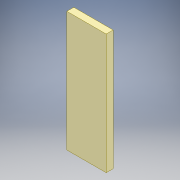
# Autodesk Inventor part: 51单片机
Saved by Autodesk Inventor 2018 (Build 220112000, 112)
## iProperties
Created: 2020-11-25
Part Number: 51单片机
Material: 尼龙 6/6
Document SubType Name: Modeling
Designer: OHHHHHHHHHH
Density: 1.13 g/cm^3
Appearance: 尼龙 6
Author: OHHHHHHHHHH
Autodesk Inventor part; units mm, degrees
ref_plane "YZ Plane" through (0, 0, 0) normal (1, 0, 0) x (0, 1, 0)
ref_plane "XZ Plane" through (0, 0, 0) normal (0, 1, 0) x (-1, 0, 0)
ref_plane "XY Plane" through (0, 0, 0) normal (0, 0, 1) x (1, 0, 0)
sketch "草图1" plane through (0, 0, 0) normal (0, 1, 0) x (-1, 0, 0)
  line L0 (0, 0) -> (17, 0)
  line L1 (17, 0) -> (17, -52)
  line L2 (17, -52) -> (0, -52)
  line L3 (0, -52) -> (0, 0)
  dimension "d0" = 52
  dimension "d1" = 17
  constraints: 8 end point, 2 parallel, 1 horizontal, 1 perpendicular
  measures "d0" distance of L0.end L1.end
  measures "d1" distance of L0.start L0.end
extrude "拉伸1" add sketch "草图1" along normal blind 3
sketch "草图2" plane through (0, 3, 0) normal (0, 1, 0) x (1, 0, 0)
  line L0 (-8.4489, 20.8819) -> (-3.8745, 20.8819) construction
  line L1 (-3.8745, 20.8819) -> (-3.8745, 17.7598) construction
  line L2 (-3.8745, 17.7598) -> (-8.4489, 17.7598) construction
  line L3 (-8.4489, 17.7598) -> (-8.4489, 20.8819) construction
  constraints: 2 other
